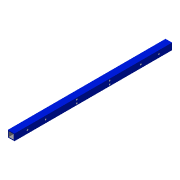
# Autodesk Inventor part: clawBase
Saved by Autodesk Inventor 2015 (Build 190159000, 159)
## iProperties
Created: 2015-01-13
Part Number: clawBase
Material: Generic
Document SubType Name: Modeling
Designer: Collin_2
Density: 1 g/cm^3
Appearance: Default
Author: Collin_2
Autodesk Inventor part; units mm, degrees
ref_plane "YZ Plane" through (0, 0, 0) normal (1, 0, 0) x (0, 1, 0)
ref_plane "XZ Plane" through (0, 0, 0) normal (0, 1, 0) x (-1, 0, 0)
ref_plane "XY Plane" through (0, 0, 0) normal (0, 0, 1) x (1, 0, 0)
sketch "Sketch1" plane through (0, 0, 0) normal (0, 1, 0) x (-1, 0, 0)
  line L0 (49.7782, 121.4529) -> (24.3782, 121.4529)
  line L1 (24.3782, 121.4529) -> (24.3782, -488.1471)
  line L2 (24.3782, -488.1471) -> (49.7782, -488.1471)
  line L3 (49.7782, -488.1471) -> (49.7782, 121.4529)
  point P0 (0, 0)
  dimension "d0" = 25.4
  dimension "d1" = 609.6
  constraints: 8 end point, 2 parallel, 1 horizontal, 1 perpendicular
  measures "d0" distance of L0.start L0.end
  measures "d1" distance of L2.end L0.start
extrude "Extrusion1" add sketch "Sketch1" along normal blind 25.4
sketch "Sketch2" plane through (-49.7782, 0, 121.4529) normal (0, 0, 1) x (1, 0, 0)
  line L0 (0, 25.4) -> (25.4, 25.4)
  line L1 (25.4, 25.4) -> (25.4, 0)
  line L2 (25.4, 0) -> (0, 0)
  line L3 (0, 0) -> (0, 25.4)
  line L4 (3.175, 22.225) -> (22.225, 22.225)
  line L5 (22.225, 22.225) -> (22.225, 3.175)
  line L6 (22.225, 3.175) -> (3.175, 3.175)
  line L7 (3.175, 3.175) -> (3.175, 22.225)
  point P0 (49.7782, 0)
  dimension "d5" = 3.175
  dimension "d6" = 3.175
  dimension "d7" = 3.175
  dimension "d8" = 3.175
  constraints: 16 end point, 4 parallel, 2 horizontal, 2 perpendicular
  measures "d5" distance between parallel lines of L1 L5
  measures "d6" distance between parallel lines of L3 L7
  measures "d7" distance between parallel lines of L0 L4
  measures "d8" distance between parallel lines of L2 L6
extrude "Extrusion2" cut sketch "Sketch2" against normal blind 508 contours L4 L5 L6 L7
sketch "Sketch3" plane through (-24.3782, 0, 121.4529) normal (1, 0, 0) x (0, 0, -1)
  circle A0 centre (241.3, 19.05) radius 3.175
  circle A1 centre (241.3, 6.35) radius 3.175
  line L0 (0, 25.4) -> (609.6, 25.4) projected
  line L1 (0, 0) -> (0, 25.4) projected
  line L2 (304.8, 25.4) -> (304.8, 0) construction
  circle A2 centre (368.3, 19.05) radius 3.175
  circle A3 centre (368.3, 6.35) radius 3.175
  point P0 (121.4529, 0)
  dimension "d11" = 6.35
  dimension "d12" = 6.35
  dimension "d14" = 12.7
  dimension "d15" = 6.35
  dimension "d26" = 304.8
  dimension "d27" = 63.5
  dimension "d28" = 63.5
  constraints: 4 centre point, 2 end point, 2 symmetric about line, 1 midpoint, 1 vertical, 2 other
  measures "d11" diameter of A0
  measures "d12" diameter of A1
  measures "d14" distance of A1.centre A0.centre
  measures "d15" distance from line of L0 A0.centre
  measures "d26" distance between parallel lines of L1 L2
  measures "d27" distance from line of L2 A0.centre
  measures "d28" distance from line of L2 A1.centre
extrude "Extrusion3" cut sketch "Sketch3" against normal blind 12.7
sketch "Sketch4" plane through (-24.3782, 0, 121.4529) normal (1, 0, 0) x (0, 0, -1)
  line L0 (0, 25.4) -> (609.6, 25.4) construction
  line L1 (304.8, 25.4) -> (304.8, 0) construction
  line L2 (0, 0) -> (0, 25.4) construction
  line L3 (120.65, 25.4) -> (120.65, 0) construction
  circle A0 centre (120.65, 12.7) radius 3.175
  circle A1 centre (488.95, 12.7) radius 3.175
  point P0 (121.4529, 0)
  dimension "d20" = 304.8
  dimension "d21" = 184.15
  dimension "d22" = 6.35
  dimension "d23" = 12.7
  constraints: 4 end point, 2 centre point, 2 midpoint, 1 perpendicular, 1 point on line, 1 symmetric about line, 1 vertical, 1 other
  measures "d20" distance between parallel lines of L1 L2
  measures "d21" distance between parallel lines of L3 L1
  measures "d22" diameter of A0
  measures "d23" distance of L3.start A0.centre
extrude "Extrusion4" cut sketch "Sketch4" against normal blind 25.4
sketch "Sketch6" plane through (-24.3782, 0, 121.4529) normal (1, 0, 0) x (0, 0, -1)
  line L0 (0, 0) -> (609.6, 0) projected
  line L1 (304.8, 0) -> (304.8, 25.4)
  line L2 (0, 25.4) -> (609.6, 25.4) projected
  line L3 (0, 0) -> (0, 25.4) projected
  circle A0 centre (50.8, 12.7) radius 3.175
  circle A1 centre (558.8, 12.7) radius 3.175
  point P0 (121.4529, 0)
  dimension "d29" = 304.8
  dimension "d30" = 6.35
  dimension "d31" = 12.7
  dimension "d32" = 254
  constraints: 2 centre point, 2 end point, 2 midpoint, 1 symmetric about line, 1 other
  measures "d29" distance between parallel lines of L3 L1
  measures "d30" diameter of A0
  measures "d31" distance from line of L0 A0.centre
  measures "d32" distance from line of A0.centre L1
extrude "Extrusion5" cut sketch "Sketch6" against normal blind 25.4 contours A0 | A1
body "Solid1"
